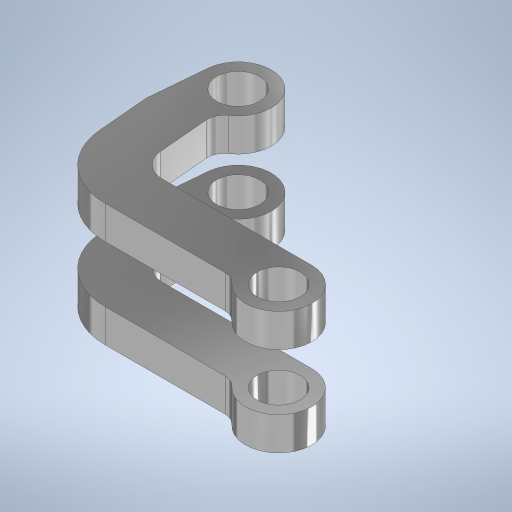
# Autodesk Inventor part: D26 Linkages
Saved by Autodesk Inventor 2024 (Build 280153000, 153)
## iProperties
Created: 2007-06-13
Part Number: D26 Linkages
Material: Steel
Description: Linkage
Document SubType Name: Modeling
Designer: G.K.
Authority: Design by UAB Čeli APS
Mass: 0.988903 g
Surface Area: 2.62623 cm^2
Volume: 0.125975 cm^3
Density: 7.85 g/cm^3
Appearance: Chrome - Polished
Mase: 0.0009889
Autodesk Inventor part; units mm, degrees
ref_plane "YZ Plane" through (0, 0, 0) normal (1, 0, 0) x (0, 1, 0)
ref_plane "XZ Plane" through (0, 0, 0) normal (0, 1, 0) x (-1, 0, 0)
ref_plane "XY Plane" through (0, 0, 0) normal (0, 0, 1) x (1, 0, 0)
sketch "Sketch1" plane through (0, 0, 0) normal (0, 0, 1) x (1, 0, 0)
  line L0 (-16.4974, 0) -> (7.0477, 0) projected
  arc A0 (-9.2978, 7.5831) -> (-12.3954, 9.4243) centre (-10.403, 9.25) ccw
  arc A1 (-0.4489, -1.0833) -> (1.0419, 2.25) centre (1.0419, 0.25) ccw
  line L1 (-12.3954, 9.4243) -> (-12.6949, 6)
  line L2 (-12.6949, 6) -> (-12.4238, 2.9014)
  line L3 (-9.7414, 6.6625) -> (-9.4752, 3.6193)
  line L4 (-7.9809, 2.25) -> (1.0419, 2.25)
  line L5 (-1.1942, -0.75) -> (-8.4391, -0.75)
  arc A2 (-9.2978, 7.5831) -> (-9.7414, 6.6625) centre (-8.7452, 6.7496) ccw
  arc A3 (-9.4752, 3.6193) -> (-7.9809, 2.25) centre (-7.9809, 3.75) ccw
  arc A4 (-12.4238, 2.9014) -> (-8.4391, -0.75) centre (-8.4391, 3.25) ccw
  arc A5 (-0.4489, -1.0833) -> (-1.1942, -0.75) centre (-1.1942, -1.75) ccw
  circle A6 centre (-10.403, 9.25) radius 1.3
  circle A7 centre (1.0419, 0.25) radius 1.3
  line L6 (-10.403, 9.25) -> (1.0419, 0.25) construction
  point P0 (0, 0)
  dimension "d4" = 3
  dimension "d5" = 4
  dimension "d6" = 3
  dimension "d13" = 6
  dimension "d15" = 1
  dimension "d16" = 1.5
  dimension "d17" = 4
  dimension "d18" = 1
  dimension "d27" = 10
  dimension "d31" = 95
  dimension "d32" = 2.6
  dimension "d34" = 0.75
  dimension "d39" = 7
  dimension "d41" = 11.4448
  constraints: 13 end point, 12 point on circle, 10 tangent, 8 centre point, 2 coincident, 2 equal radius, 2 parallel, 1 horizontal
  measures "d4" distance between parallel lines of L3 L2
  measures "d5" diameter of A0
  measures "d6" distance between parallel lines of L5 L4
  measures "d13" distance from line of L0 L1.end
  measures "d15" radius of A2
  measures "d16" radius of A3
  measures "d17" radius of A4
  measures "d18" radius of A5
  measures "d27" angle of L2 L1
  measures "d31" angle of L4 L3
  measures "d32" diameter of A6
  measures "d34" distance between parallel lines of L0 L5
  measures "d39" distance from line of L6.start L4
  measures "d41" horizontal distance of L6.start A1.centre
extrude "Extrusion1" add sketch "Sketch1" along normal blind 2 contours A4 L2 L1 A0 A2 L3 A3 L4 A1 L0 A7 | L0 A7 A1 A5 L5 A4
pattern_linear "Rectangular Pattern1" count 2 spacing 5.4 along (0, 0, 1)
body "Solid1"
